Axe 3 (Autodesk Fusion 360 design; units mm, degrees)
Autodesk Fusion 360 part; units mm, degrees
sketch "Sketch1" plane through (0, 0, 0) normal (0, 0, 1) x (1, 0, 0)
  circle A0 centre (0, 0) radius 9
  circle A1 centre (0, 0) radius 2.1
  dimension "d1" = 18
  dimension "d25" = 4.2
  constraint coincident A0.centre A1.centre
  measures "d1" diameter of A0
  measures "d25" diameter of A1
extrude "Extrude1" add sketch "Sketch1" against normal blind 1.5
sketch "Sketch2" plane through (0, 0, -1.5) normal (0, 0, -1) x (1, 0, 0)
  circle A0 centre (0, 0) radius 9
  circle A1 centre (0, 0) radius 8
  circle A2 centre (0, 0) radius 2.1
  dimension "d10" = 16
  constraint concentric A0 A1
  measures "d10" diameter of A1
extrude "Extrude3" add sketch "Sketch2" along normal blind 0.5 contours A1
sketch "Sketch3" plane through (0, 0, -2) normal (0, 0, -1) x (1, 0, 0)
  circle A0 centre (0, 0) radius 6
  circle A1 centre (0, 0) radius 8
  circle A2 centre (0, 0) radius 2.1
  dimension "d13" = 12
  constraint coincident A0.centre A1.centre
  measures "d13" diameter of A0
extrude "Extrude4" add sketch "Sketch3" along normal blind 3.5 contours A0
sketch "Sketch4" plane through (0, 0, -5.5) normal (0, 0, -1) x (1, 0, 0)
  circle A0 centre (0, 0) radius 6
  line L0 (-1.963, 3.4) -> (-3.926, 0)
  line L1 (-3.926, 0) -> (-1.963, -3.4)
  line L2 (-1.963, -3.4) -> (1.963, -3.4)
  line L3 (1.963, -3.4) -> (3.926, 0)
  line L4 (3.926, 0) -> (1.963, 3.4)
  line L5 (1.963, 3.4) -> (-1.963, 3.4)
  circle A1 centre (0, 0) radius 2.1
  dimension "d24" = 6.8
  constraint coincident A0.centre A1.centre
  measures "d24" distance of L2 L5
extrude "Extrude5" add sketch "Sketch4" along normal blind 16 contours L0 L1 L2 L3 L4 L5
named bodies: "Axe3"
